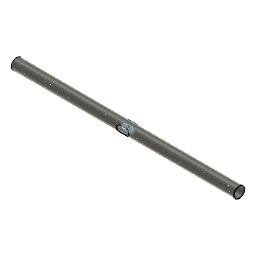
tube+carbone (Autodesk Fusion 360 design; units mm, degrees)
Autodesk Fusion 360 part; units mm, degrees
sketch "Sketch1" plane through (0, 0, 0) normal (1, 0, 0) x (0, 1, 0)
  circle A0 centre (0, 0) radius 12.5
  circle A1 centre (0, 0) radius 11.5
  dimension "d2" = 25
  dimension "d3" = 23
  constraint concentric A0 A1
  constraint coincident A0.centre A1.centre
  measures "d2" diameter of A0
  measures "d3" diameter of A1
extrude "Extrude1" add sketch "Sketch1" along normal blind 500
sketch "Sketch4" plane through (0, 0, 0) normal (0, 1, 0) x (1, 0, 0)
  arc A0 (243, 7) -> (243, -7) centre (243, 0) ccw
  arc A1 (257, -7) -> (257, 7) centre (257, 0) ccw
  line L0 (243, 7) -> (257, 7)
  line L1 (257, -7) -> (243, -7)
  constraint tangent A1 L0
  constraint tangent A0 L1
extrude "Extrude2" cut sketch "Sketch4" along normal blind 444
extrude "Extrude3" cut sketch "Sketch4" against normal blind 41
